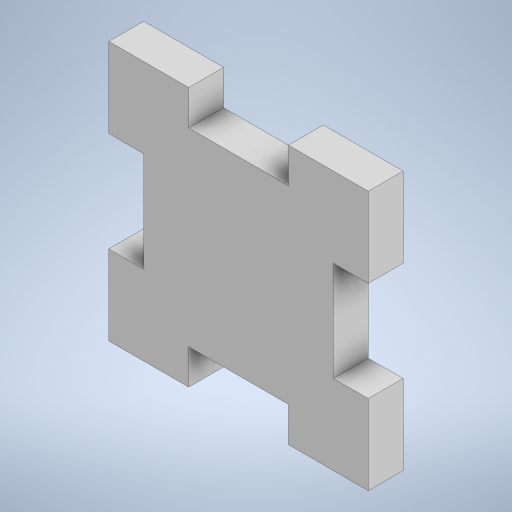
# Autodesk Inventor part: Spodi Spodnji
Saved by Autodesk Inventor 2023 (Build 270158000, 158)
## iProperties
Created: 2022-12-19
Part Number: Spodi Spodnji
Material: Generic
Document SubType Name: Modeling
Designer: David Zindović
Density: 1 g/cm^3
Appearance: Default
Author: David Zindović
Autodesk Inventor part; units mm, degrees
ref_plane "YZ Plane" through (0, 0, 0) normal (1, 0, 0) x (0, 1, 0)
ref_plane "XZ Plane" through (0, 0, 0) normal (0, 1, 0) x (-1, 0, 0)
ref_plane "XY Plane" through (0, 0, 0) normal (0, 0, 1) x (1, 0, 0)
sketch "Sketch1" plane through (0, 0, 0) normal (0, 0, 1) x (1, 0, 0)
  circle A0 centre (0, 0) radius 6
  line L0 (-13, 13) -> (13, 13)
  line L1 (13, 13) -> (13, -13)
  line L2 (13, -13) -> (-13, -13)
  line L3 (-13, -13) -> (-13, 13)
  line L4 (0, 0) -> (13, 13)
  line L5 (6.5, 6.5) -> (13, 13)
  circle A1 centre (9.75, 9.75) radius 0.5
  line L6 (0, 0) -> (-13, 13)
  line L7 (-6.5, 6.5) -> (-13, 13)
  circle A2 centre (-9.75, 9.75) radius 0.5
  line L8 (0, 0) -> (-13, -13)
  line L9 (-6.5, -6.5) -> (-13, -13)
  circle A3 centre (-9.75, -9.75) radius 0.5
  line L10 (0, 0) -> (13, -13)
  line L11 (6.5, -6.5) -> (13, -13)
  circle A4 centre (9.75, -9.75) radius 0.5
  line L12 (-5, -13) -> (5, -13)
  line L13 (5, -13) -> (5, -9.5)
  line L14 (5, -9.5) -> (-5, -9.5)
  line L15 (-5, -9.5) -> (-5, -13)
  line L16 (13, 5) -> (9.5, 5)
  line L17 (9.5, 5) -> (9.5, -5)
  line L18 (9.5, -5) -> (13, -5)
  line L19 (-5, 13) -> (-5, 9.5)
  line L20 (-5, 9.5) -> (5, 9.5)
  line L21 (5, 9.5) -> (5, 13)
  line L22 (-13, -5) -> (-9.5, -5)
  line L23 (-9.5, -5) -> (-9.5, 5)
  line L24 (-9.5, 5) -> (-13, 5)
  point P0 (0, 13)
  point P1 (13, 0)
  point P2 (0, -9.5)
  point P3 (0, -13)
  point P4 (9.5, 0)
  point P5 (0, 9.5)
  point P6 (-9.5, 0)
  dimension "d4" = 12
  dimension "d5" = 26
  dimension "d6" = 26
  dimension "d7" = 1
  dimension "d8" = 360
  dimension "d9" = 10
  dimension "d10" = 3.5
  dimension "d11" = 360
  constraints: 50 end point, 6 midpoint, 5 centre point, 4 parallel, 2 horizontal, 2 perpendicular, 2 vertical alignment, 1 coincident, 1 collinear, 1 horizontal alignment, 1 point on line, 62 other
  measures "d4" diameter of A0
  measures "d5" distance of L0.start L0.end
  measures "d6" distance of L0.end L1.end
  measures "d7" diameter of A1
  measures "d9" distance of L14.end L13.end
  measures "d10" distance of L12.end L13.end
extrude "Extrusion1" add sketch "Sketch1" along normal mid plane 3.5 contours A0 L10 L4 | A0 L4 A1 L1 L16 L17 L18 L10 A4 | L4 L6 A0 | A0 L6 A2 L0 L19 L20 L21 L4 A1 | L10 A4 L2 L13 L14 L15 L8 A3 A0 | A0 L8 L10 | L6 L8 A0 | A0 L8 A3 L3 L22 L23 L24 L6 A2 | A1 L4 | L4 A1 | A4 L10 | L10 A4 | A2 L6 | L6 A2 | A3 L8 | L8 A3
equation "\"d6\" = d5"
body "Solid1"
